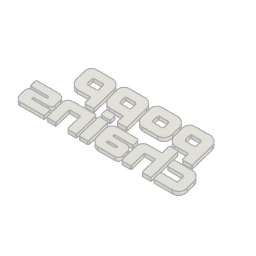
3PoppChains Logo (Autodesk Fusion 360 design; units mm, degrees)
Autodesk Fusion 360 part; units mm, degrees
sketch "PoppChains Logo back" plane through (0, 0, 0) normal (0, 0, 1) x (1, 0, 0)
  line L0 (-12.7934, 7.4385) -> (-14.8073, 7.4385)
  line L1 (-18.0622, -4.0245) -> (-18.1371, -3.7245)
  line L2 (15.775, -3.4869) -> (12.3633, -3.4869)
  line L3 (12.0442, -2.2702) -> (15.4711, -2.2702)
  line L4 (15.4711, -2.2702) -> (15.775, -3.4869)
  arc A0 (11.7104, -2.1972) -> (12.0442, -2.2702) centre (12.0442, -1.4702) ccw
  line L5 (12.0584, -3.5906) -> (11.7104, -2.1972)
  arc A1 (12.3633, -3.4869) -> (12.0584, -3.5906) centre (12.3633, -3.9869) ccw
  spline S0 degree 3 poles (-8.9047, 3.9854) (-8.8081, 3.8641) (-8.7015, 3.7457) (-8.5857, 3.6335) (-8.1655, 3.2264) (-7.6733, 2.9494) (-7.2518, 2.8544) knots 0.109065 0.109065 0.109065 0.109065 0.144103 0.144103 0.144103 0.271229 0.271229 0.271229 0.271229
  spline S1 degree 3 poles (-8.5032, 9.9808) (-9.0129, 9.9808) (-9.5792, 9.7861) (-9.9156, 9.3575) (-10.1073, 9.1132) (-10.2067, 8.8146) (-10.2332, 8.5124) knots 0 0 0 0 0.118832 0.118832 0.118832 0.186572 0.186572 0.186572 0.186572
  spline S2 degree 3 poles (-8.2671, 1.4319) (-8.2484, 1.3571) (-8.211, 1.2855) (-8.27, 1.1136) (-8.3064, 1.0076) (-8.4409, 0.8691) (-8.5685, 0.8357) (-8.6104, 0.8247) (-8.6486, 0.8212) (-8.6817, 0.8212) knots 0 0 0 0 0.007204 0.007204 0.007204 0.011648 0.011648 0.011648 0.01311 0.01311 0.01311 0.01311
  spline S3 degree 2 poles (-12.3757, 7.1783) (-12.4406, 7.4385) (-12.7934, 7.4385) knots 0 0 0 0.053563 0.053563 0.053563 weights 1 1.286007 1
  line L6 (-6.5576, 5.9139) -> (-6.8384, 7.0385)
  line L7 (1.7578, -4.1644) -> (-0.2132, -4.1644)
  arc A2 (-0.4322, -3.9129) -> (-0.2381, -3.6644) centre (-0.2381, -3.8644) cw
  line L8 (-0.4072, -4.0129) -> (-0.4322, -3.9129)
  line L9 (-0.2381, -3.6644) -> (1.7328, -3.6644)
  arc A3 (1.9518, -3.9159) -> (1.7578, -4.1644) centre (1.7578, -3.9644) cw
  arc A4 (-0.2132, -4.1644) -> (-0.4072, -4.0129) centre (-0.2132, -3.9644) cw
  line L10 (1.9268, -3.8159) -> (1.9518, -3.9159)
  arc A5 (1.7328, -3.6644) -> (1.9268, -3.8159) centre (1.7328, -3.8644) cw
  spline S4 degree 2 poles (-16.2032, 9.5808) (-17.8989, 9.5808) (-17.4933, 7.9566) knots 0 0 0 0.236399 0.236399 0.236399 weights 1 0.745447 1
  spline S5 degree 2 poles (-14.3421, 5.4627) (-14.5571, 5.4627) (-14.6454, 5.8161) knots 0 0 0 0.047921 0.047921 0.047921 weights 1 0.521199 1
  arc A6 (-7.2518, 2.8544) -> (-7.4125, 2.3527) centre (-6.9274, 2.4738) ccw
  arc A7 (-4.4905, 5.4627) -> (-4.3062, 5.6987) centre (-4.4905, 5.6527) ccw
  line L11 (-12.4594, 5.8627) -> (-14.2298, 5.8627)
  arc A8 (-11.3768, 3.1416) -> (-11.4739, 3.2173) centre (-11.4739, 3.1173) ccw
  spline S6 degree 2 poles (-20.0623, -2.1426) (-20.9037, -2.1426) (-20.6795, -3.0405) knots 0 0 0 0.121296 0.121296 0.121296 weights 1 0.623284 1
  spline S7 degree 2 poles (-0.9081, 1.3468) (-0.8767, 1.2212) (-0.9817, 1.2212) knots 0 0 0 0.017347 0.017347 0.017347 weights 1 1.074969 1
  spline S8 degree 2 poles (-9.1042, 5.197) (-8.6099, 3.2173) (-6.9332, 3.2173) knots 0 0 0 0.304949 0.304949 0.304949 weights 1 0.564634 1
  line L12 (-2.8716, -6.5063) -> (-4.5755, -6.5063)
  line L13 (-14.6332, 2.8173) -> (-11.7081, 2.8173)
  arc A9 (-6.7172, 0.4953) -> (-6.7594, 0.4425) centre (-6.3489, 0.1571) ccw
  line L14 (-14.2576, 5.9139) -> (-14.5384, 7.0385)
  line L15 (-12.1905, 5.4627) -> (-14.3421, 5.4627)
  line L16 (-12.4594, 5.8627) -> (-12.7528, 7.0377)
  spline S9 degree 3 poles (-12.7528, 7.0377) (-12.7645, 7.0382) (-12.7779, 7.0385) (-12.7934, 7.0385) knots 0.049882 0.049882 0.049882 0.049882 0.053563 0.053563 0.053563 0.053563
  line L17 (-12.0062, 5.6987) -> (-12.3757, 7.1783)
  arc A10 (-8.6888, -1.9459) -> (-8.7858, -1.8702) centre (-8.7858, -1.9702) ccw
  line L18 (-14.6454, 5.8161) -> (-14.9916, 7.2025)
  arc A11 (-16.5004, -2.1426) -> (-16.4034, -2.0184) centre (-16.5004, -2.0426) ccw
  spline S10 degree 3 poles (-0.52, 1.4437) (-0.4968, 1.3508) (-0.4654, 1.2156) (-0.5661, 1.0465) (-0.6478, 0.9093) (-0.8137, 0.8366) (-0.9176, 0.8248) (-0.9404, 0.8222) (-0.9616, 0.8212) (-0.9817, 0.8212) knots 0 0 0 0 0.008721 0.008721 0.008721 0.015794 0.015794 0.015794 0.017347 0.017347 0.017347 0.017347
  spline S11 degree 3 poles (-16.2032, 9.9808) (-16.7129, 9.9808) (-17.2792, 9.7861) (-17.6156, 9.3575) (-17.9484, 8.9335) (-18.0028, 8.3459) (-17.8814, 7.8597) knots 0 0 0 0 0.118832 0.118832 0.118832 0.236399 0.236399 0.236399 0.236399
  line L19 (-2.6776, -5.8579) -> (-4.1289, -0.046)
  line L20 (-6.4459, 0.1329) -> (-4.9636, -5.8032)
  arc A12 (-4.9636, -5.8032) -> (-4.5755, -6.1063) centre (-4.5755, -5.7063) ccw
  arc A13 (-2.8716, -6.1063) -> (-2.6776, -5.8579) centre (-2.8716, -5.9063) ccw
  line L21 (-4.5755, -6.1063) -> (-2.8716, -6.1063)
  arc A14 (-6.3489, 0.2571) -> (-6.4459, 0.1329) centre (-6.3489, 0.1571) ccw
  arc A15 (-4.1289, -0.046) -> (-4.517, 0.2571) centre (-4.517, -0.1429) ccw
  line L22 (-4.517, 0.2571) -> (-6.3489, 0.2571)
  line L23 (-3.2543, -1.367) -> (-2.5651, -4.1266)
  arc A16 (-0.8552, -1.6474) -> (-0.9523, -1.7717) centre (-0.8552, -1.7474) ccw
  spline S12 degree 2 poles (-1.9641, 0.2571) (-3.6598, 0.2571) (-3.2543, -1.367) knots 0 0 0 0.236399 0.236399 0.236399 weights 1 0.745447 1
  spline S13 degree 3 poles (-2.4089, -5.2829) (-2.3011, -5.4235) (-2.18, -5.5609) (-2.0466, -5.6902) (-1.555, -6.1665) (-0.9648, -6.4646) (-0.5045, -6.5018) (-0.4671, -6.5048) (-0.4302, -6.5063) (-0.3941, -6.5063) knots 0.103755 0.103755 0.103755 0.103755 0.144103 0.144103 0.144103 0.292842 0.292842 0.292842 0.304949 0.304949 0.304949 0.304949
  spline S14 degree 3 poles (-10.6898, 0.8212) (-10.9685, 0.8212) (-11.1444, 0.9908) (-11.2604, 1.1724) (-11.2987, 1.2322) (-11.3282, 1.2957) (-11.3458, 1.3662) knots 0 0 0 0 0.028075 0.028075 0.028075 0.037327 0.037327 0.037327 0.037327
  line L24 (-13.7235, -1.3469) -> (-12.6106, -5.8032)
  arc A17 (-20.89, -1.5668) -> (-20.793, -1.6426) centre (-20.793, -1.5426) ccw
  line L25 (-4.7594, 5.8627) -> (-6.5298, 5.8627)
  line L26 (-0.9523, -1.7717) -> (-0.9341, -1.8444)
  arc A18 (-12.6106, -5.8032) -> (-12.2225, -6.1063) centre (-12.2225, -5.7063) ccw
  arc A19 (-2.8716, -6.5063) -> (-2.2895, -5.761) centre (-2.8716, -5.9063) ccw
  arc A20 (-5.5313, -6.5063) -> (-5.1207, -6.2917) centre (-5.5313, -6.0063) ccw
  line L27 (-20.89, -1.5668) -> (-21.3145, 0.1329)
  spline S15 degree 3 poles (-12.5141, 0.6571) (-13.0001, 0.6571) (-13.5417, 0.4643) (-13.8613, 0.0466) (-13.9756, -0.1028) (-14.0554, -0.2722) (-14.1056, -0.4501) knots 0 0 0 0 0.113726 0.113726 0.113726 0.154398 0.154398 0.154398 0.154398
  arc A21 (-11.2381, -1.8702) -> (-11.3352, -1.9944) centre (-11.2381, -1.9702) ccw
  line L28 (-5.0934, 7.0385) -> (-6.8384, 7.0385)
  line L29 (-2.4089, -5.2829) -> (-2.2895, -5.761)
  spline S16 degree 3 poles (-20.7806, -2.0426) (-20.841, -2.1031) (-20.8961, -2.1737) (-20.941, -2.2484) (-21.1119, -2.5324) (-21.1327, -2.8768) (-21.0676, -3.1375) knots 0.049481 0.049481 0.049481 0.049481 0.064439 0.064439 0.064439 0.121296 0.121296 0.121296 0.121296
  line L30 (-13.8926, -2.7331) -> (-14.3478, -0.9104)
  arc A22 (-5.1207, -6.2917) -> (-4.5755, -6.5063) centre (-4.5755, -5.7063) ccw
  line L31 (-17.8814, 7.8597) -> (-17.1923, 5.1001)
  line L32 (-6.9332, 3.2173) -> (-3.7739, 3.2173)
  arc A23 (-13.1783, -6.1063) -> (-13.0813, -5.9821) centre (-13.1783, -6.0063) ccw
  arc A24 (-18.0401, -3.6003) -> (-18.1371, -3.7245) centre (-18.0401, -3.7003) ccw
  arc A25 (-0.9341, -1.8444) -> (-0.546, -2.1474) centre (-0.546, -1.7474) ccw
  line L33 (-5.4343, -5.9821) -> (-6.9166, -0.046)
  arc A26 (-21.2175, 0.2571) -> (-21.3145, 0.1329) centre (-21.2175, 0.1571) ccw
  arc A27 (-13.4755, -4.4033) -> (-13.8636, -4.1003) centre (-13.8636, -4.5003) ccw
  line L34 (-3.7408, 0.0509) -> (-3.6199, -0.4335)
  arc A28 (-21.2175, 0.6571) -> (-21.7026, 0.036) centre (-21.2175, 0.1571) ccw
  line L35 (-13.0813, -5.9821) -> (-13.4755, -4.4033)
  arc A29 (-12.7678, -6.2917) -> (-12.2225, -6.5063) centre (-12.2225, -5.7063) ccw
  line L36 (-5.5313, -6.1063) -> (-7.3375, -6.1063)
  spline S17 degree 2 poles (-2.5651, -4.1266) (-2.0708, -6.1063) (-0.3941, -6.1063) knots 0 0 0 0.304949 0.304949 0.304949 weights 1 0.564634 1
  line L37 (-12.7934, 7.0385) -> (-14.5384, 7.0385)
  arc A30 (-13.1783, -6.5063) -> (-12.7678, -6.2917) centre (-13.1783, -6.0063) ccw
  spline S18 degree 2 poles (-14.3478, -0.9104) (-14.6393, 0.2571) (-15.8774, 0.2571) knots 0 0 0 0.201598 0.201598 0.201598 weights 1 0.666667 1
  line L38 (-16.4783, -1.7184) -> (-16.4034, -2.0184)
  line L39 (8.7039, -2.2702) -> (9.6435, -6.033)
  spline S19 degree 3 poles (7.8687, -5.8354) (7.8948, -5.9397) (7.9271, -6.0356) (7.8693, -6.2046) (7.8256, -6.3322) (7.6744, -6.469) (7.5501, -6.503) (7.4957, -6.5179) (7.4481, -6.5217) (7.4054, -6.5217) knots 0 0 0 0 0.011564 0.011564 0.011564 0.020294 0.020294 0.020294 0.024116 0.024116 0.024116 0.024116
  spline S20 degree 2 poles (6.4947, -1.9838) (6.4663, -1.8702) (6.5435, -1.8702) knots 0 0 0 0.014326 0.014326 0.014326 weights 1 0.986543 1
  line L40 (7.4054, -6.5217) -> (5.4872, -6.5217)
  arc A31 (8.361, 0.2571) -> (8.458, 0.3813) centre (8.361, 0.3571) ccw
  line L41 (6.4947, -1.9838) -> (7.4806, -5.9323)
  arc A32 (9.6435, -6.033) -> (10.2741, -6.5255) centre (10.2741, -5.8755) ccw
  line L42 (9.0447, -1.9838) -> (10.0316, -5.9361)
  spline S21 degree 2 poles (7.4806, -5.9323) (7.528, -6.1217) (7.4054, -6.1217) knots 0 0 0 0.024116 0.024116 0.024116 weights 1 1.205865 1
  line L43 (7.4054, -6.1217) -> (5.4872, -6.1217)
  arc A33 (10.0316, -5.9361) -> (10.2741, -6.1255) centre (10.2741, -5.8755) ccw
  line L44 (6.9784, -2.2702) -> (7.8687, -5.8354)
  spline S22 degree 2 poles (6.4316, 5.2185) (6.9313, 3.2173) (8.5168, 3.2173) knots 0 0 0 0.299728 0.299728 0.299728 weights 1 0.564634 1
  arc A34 (8.3427, 7.4385) -> (8.1584, 7.2025) centre (8.3427, 7.2485) ccw
  line L45 (5.7425, 7.9781) -> (6.4316, 5.2185)
  line L46 (10.3566, 7.0385) -> (8.6116, 7.0385)
  line L47 (10.6906, 5.8627) -> (10.3972, 7.0377)
  spline S23 degree 2 poles (8.8079, 5.4627) (8.5929, 5.4627) (8.5046, 5.8161) knots 0 0 0 0.047921 0.047921 0.047921 weights 1 0.521199 1
  arc A35 (7.8936, 2.9606) -> (7.5515, 2.3603) centre (8.0366, 2.4815) ccw
  line L48 (10.3566, 7.4385) -> (8.3427, 7.4385)
  line L49 (8.0366, 2.5815) -> (9.7924, 2.5815)
  spline S24 degree 3 poles (6.3587, 4.3835) (6.509, 4.1271) (6.7031, 3.8674) (6.9338, 3.6346) (7.2352, 3.3306) (7.5726, 3.0983) (7.8936, 2.9606) knots 0.071956 0.071956 0.071956 0.071956 0.14301 0.14301 0.14301 0.235825 0.235825 0.235825 0.235825
  line L50 (10.6906, 5.8627) -> (8.9202, 5.8627)
  spline S25 degree 2 poles (6.9468, 9.5808) (5.3423, 9.5808) (5.7425, 7.9781) knots 0 0 0 0.228466 0.228466 0.228466 weights 1 0.745447 1
  line L51 (8.8924, 5.9139) -> (8.6116, 7.0385)
  line L52 (8.5046, 5.8161) -> (8.1584, 7.2025)
  arc A36 (10.5686, 2.3753) -> (10.2779, 2.8173) centre (9.7924, 2.1815) ccw
  arc A37 (10.1805, 2.2784) -> (9.7924, 2.5815) centre (9.7924, 2.1815) ccw
  spline S26 degree 3 poles (10.3972, 7.0377) (10.3855, 7.0382) (10.3721, 7.0385) (10.3566, 7.0385) knots 0.049882 0.049882 0.049882 0.049882 0.053563 0.053563 0.053563 0.053563
  spline S27 degree 3 poles (8.9202, 5.8627) (8.9047, 5.885) (8.8943, 5.9083) (8.8924, 5.9139) knots 0.029456 0.029456 0.029456 0.029456 0.044721 0.044721 0.044721 0.044721
  spline S28 degree 3 poles (6.3587, 4.3835) (6.3212, 4.0569) (6.2153, 3.7527) (6.0237, 3.4998) (5.6676, 3.0297) (5.0602, 2.8173) (4.4476, 2.8173) knots 0.078476 0.078476 0.078476 0.078476 0.154724 0.154724 0.154724 0.296505 0.296505 0.296505 0.296505
  spline S29 degree 5 poles (5.2144, 0.2571) (5.2086, 0.2571) (5.1964, 0.2572) (5.1763, 0.2578) (5.1458, 0.2592) (5.102, 0.2605) (5.0526, 0.2596) (4.9982, 0.2548) (4.9395, 0.2452) (4.8777, 0.2304) (4.814, 0.2108) (4.7496, 0.1869) (4.6858, 0.1592) (4.6237, 0.1283) (4.5643, 0.0946) (4.5084, 0.0584) (4.4562, 0.0199) (4.4081, -0.0207) (4.3635, -0.0634) (4.322, -0.1081) (4.2826, -0.1547) (4.2448, -0.2031) (4.208, -0.2532) (4.1726, -0.3046) (4.1391, -0.3569) (4.1084, -0.41) (4.0813, -0.4637) (4.0585, -0.5181) (4.0402, -0.5741) (4.0259, -0.6327) (4.0151, -0.6948) (4.0071, -0.7616) (4.0011, -0.8333) (3.9969, -0.9096) (3.9941, -0.9893) (3.9929, -1.071) (3.9934, -1.153) (3.9957, -1.2334) (4, -1.311) (4.0064, -1.3848) (4.0151, -1.4543) (4.0237, -1.5063) (4.0313, -1.5432) (4.0367, -1.5669) (4.0395, -1.5785) knots 0 0 0 0 0 0 0.025 0.05 0.075 0.1 0.125 0.15 0.175 0.2 0.225 0.25 0.275 0.3 0.325 0.35 0.375 0.4 0.425 0.45 0.475 0.5 0.525 0.55 0.575 0.6 0.625 0.65 0.675 0.7 0.725 0.75 0.775 0.8 0.825 0.85 0.875 0.9 0.925 0.95 0.975 1 1 1 1 1 1
  spline S30 degree 2 poles (5.3449, 7.5066) (4.8269, 9.5808) (2.9577, 9.5808) knots 0 0 0 0.329195 0.329195 0.329195 weights 1 0.594055 1
  spline S31 degree 3 poles (5.2144, 0.6571) (5.186, 0.6571) (4.889, 0.6635) (4.6506, 0.5763) (4.3416, 0.4633) (4.0734, 0.2363) (3.9128, 0.0202) (3.8114, -0.1163) (3.7062, -0.2874) (3.6522, -0.4818) knots 0 0 0 0 0.210086 0.210086 0.210086 0.482519 0.482519 0.482519 0.654552 0.654552 0.654552 0.654552
  spline S32 degree 3 poles (6.9468, 9.9808) (6.4622, 9.9808) (5.9221, 9.788) (5.6036, 9.371) (5.4157, 9.1249) (5.3212, 8.8246) (5.2988, 8.5214) knots 0 0 0 0 0.113417 0.113417 0.113417 0.18033 0.18033 0.18033 0.18033
  line L53 (7.9769, 0.6571) -> (7.5515, 2.3603)
  spline S33 degree 2 poles (5.8873, 5.3346) (6.416, 3.2173) (4.4476, 3.2173) knots 0 0 0 0.296505 0.296505 0.296505 weights 1 0.847333 1
  line L54 (10.6577, 9.9808) -> (6.9468, 9.9808)
  line L55 (5.8873, 5.3346) -> (5.3449, 7.5066)
  spline S34 degree 3 poles (5.2988, 8.5214) (5.1508, 8.7377) (4.9713, 8.9504) (4.7641, 9.1433) (4.2375, 9.6337) (3.5919, 9.9356) (3.0894, 9.9755) (3.0445, 9.979) (3.0006, 9.9808) (2.9577, 9.9808) knots 0.091726 0.091726 0.091726 0.091726 0.154738 0.154738 0.154738 0.314905 0.314905 0.314905 0.329195 0.329195 0.329195 0.329195
  arc A38 (4.711, -5.9157) -> (5.4872, -6.5217) centre (5.4872, -5.7217) ccw
  arc A39 (8.0366, 2.5815) -> (7.9396, 2.4572) centre (8.0366, 2.4815) ccw
  line L56 (10.6577, 9.5808) -> (6.9468, 9.5808)
  line L57 (8.458, 0.3813) -> (7.9396, 2.4572)
  line L58 (4.0395, -1.5785) -> (5.0991, -5.8187)
  line L59 (3.5001, -1.5232) -> (3.1688, -0.1974)
  spline S35 degree 3 poles (2.6972, 7.0377) (2.6855, 7.0382) (2.6721, 7.0385) (2.6566, 7.0385) knots 0.049882 0.049882 0.049882 0.049882 0.053563 0.053563 0.053563 0.053563
  spline S36 degree 2 poles (1.1079, 5.4627) (0.8929, 5.4627) (0.8046, 5.8161) knots 0 0 0 0.047921 0.047921 0.047921 weights 1 0.521199 1
  arc A40 (0.6427, 7.4385) -> (0.4584, 7.2025) centre (0.6427, 7.2485) ccw
  line L60 (3.6522, -0.4818) -> (3.5569, -0.1005)
  spline S37 degree 3 poles (1.2202, 5.8627) (1.2048, 5.8848) (1.1941, 5.9087) (1.1924, 5.9139) knots 0.029456 0.029456 0.029456 0.029456 0.044721 0.044721 0.044721 0.044721
  line L61 (2.6566, 7.0385) -> (0.9116, 7.0385)
  spline S38 degree 3 poles (4.6962, -5.8563) (4.6582, -5.9337) (4.6125, -6.0075) (4.5584, -6.0759) (4.3359, -6.3574) (3.9893, -6.5063) (3.6964, -6.5063) knots 0.072101 0.072101 0.072101 0.072101 0.088502 0.088502 0.088502 0.156035 0.156035 0.156035 0.156035
  line L62 (2.6566, 7.4385) -> (0.6427, 7.4385)
  line L63 (3.4438, 5.6987) -> (3.0743, 7.1783)
  line L64 (0.8046, 5.8161) -> (0.4584, 7.2025)
  arc A41 (3.2595, 5.4627) -> (3.4438, 5.6987) centre (3.2595, 5.6527) ccw
  line L65 (2.5867, 0.6571) -> (-1.9641, 0.6571)
  line L66 (4.0361, -3.3747) -> (4.4167, -4.8975)
  line L67 (1.1924, 5.9139) -> (0.9116, 7.0385)
  line L68 (4.6962, -5.8563) -> (4.711, -5.9157)
  spline S39 degree 2 poles (3.0743, 7.1783) (3.0094, 7.4385) (2.6566, 7.4385) knots 0 0 0 0.053563 0.053563 0.053563 weights 1 1.286007 1
  spline S40 degree 2 poles (4.4167, -4.8975) (4.7187, -6.1063) (3.6964, -6.1063) knots 0 0 0 0.156035 0.156035 0.156035 weights 1 0.619231 1
  line L69 (3.2595, 5.4627) -> (1.1079, 5.4627)
  arc A42 (3.4031, -1.6474) -> (3.5001, -1.5232) centre (3.4031, -1.5474) ccw
  line L70 (2.9906, 5.8627) -> (2.6972, 7.0377)
  arc A43 (3.1688, -0.1974) -> (2.5867, 0.2571) centre (2.5867, -0.3429) ccw
  line L71 (2.9906, 5.8627) -> (1.2202, 5.8627)
  arc A44 (3.5569, -0.1005) -> (2.5867, 0.6571) centre (2.5867, -0.3429) ccw
  spline S41 degree 2 poles (4.0361, -3.3747) (3.7295, -2.1474) (2.492, -2.1474) knots 0 0 0 0.204563 0.204563 0.204563 weights 1 0.543429 1
  line L72 (0.8168, 2.8173) -> (4.4476, 2.8173)
  line L73 (0.8168, 3.2173) -> (4.4476, 3.2173)
  line L74 (8.7039, -2.2702) -> (6.9784, -2.2702)
  line L75 (7.9769, 0.6571) -> (5.2144, 0.6571)
  arc A45 (9.0447, -1.9838) -> (8.8991, -1.8702) centre (8.8991, -2.0202) ccw
  arc A46 (5.0991, -5.8187) -> (5.4872, -6.1217) centre (5.4872, -5.7217) ccw
  line L76 (8.361, 0.2571) -> (5.2144, 0.2571)
  line L77 (8.8991, -1.8702) -> (6.5435, -1.8702)
  line L78 (-4.0081, 2.8173) -> (-3.6458, 1.3662)
  line L79 (15.8592, -2.1733) -> (16.2561, -3.7627)
  arc A47 (11.6561, -1.5671) -> (12.0442, -1.8702) centre (12.0442, -1.4702) ccw
  line L80 (19.0529, -3.9076) -> (18.5105, -1.7355)
  line L81 (13.0276, -6.5217) -> (17.2251, -6.5217)
  line L82 (12.2662, -4.0112) -> (12.7365, -5.8944)
  arc A48 (12.7789, -6.4761) -> (13.0276, -6.5217) centre (13.0276, -5.8217) ccw
  line L83 (18.6648, -4.0045) -> (18.1224, -1.8324)
  arc A49 (15.8592, -2.1733) -> (15.4711, -1.8702) centre (15.4711, -2.2702) ccw
  spline S42 degree 2 poles (18.6648, -4.0045) (19.1935, -6.1217) (17.2251, -6.1217) knots 0 0 0 0.296505 0.296505 0.296505 weights 1 0.847333 1
  line L84 (2.9577, 9.5808) -> (-0.7532, 9.5808)
  line L85 (2.5867, 0.2571) -> (-1.9641, 0.2571)
  line L86 (-0.3941, -6.1063) -> (3.6964, -6.1063)
  line L87 (-0.3941, -6.5063) -> (3.6964, -6.5063)
  line L88 (2.9577, 9.9808) -> (-0.7532, 9.9808)
  line L89 (16.1591, -3.8869) -> (12.3633, -3.8869)
  spline S43 degree 3 poles (-1.1547, 3.9854) (-1.0581, 3.8641) (-0.9515, 3.7457) (-0.8357, 3.6335) (-0.3441, 3.1571) (0.2461, 2.8591) (0.7064, 2.8219) (0.7439, 2.8188) (0.7807, 2.8173) (0.8168, 2.8173) knots 0.109065 0.109065 0.109065 0.109065 0.144103 0.144103 0.144103 0.292842 0.292842 0.292842 0.304949 0.304949 0.304949 0.304949
  line L90 (3.4031, -1.6474) -> (-0.8552, -1.6474)
  line L91 (-0.546, -2.1474) -> (2.492, -2.1474)
  spline S44 degree 3 poles (14.9754, 1.455) (15.0011, 1.3519) (15.0173, 1.1877) (14.9096, 1.0322) (14.8062, 0.8828) (14.6427, 0.8346) (14.5375, 0.8244) (14.5134, 0.8221) (14.4906, 0.8212) (14.4683, 0.8212) knots 0 0 0 0 0.00997 0.00997 0.00997 0.019549 0.019549 0.019549 0.021738 0.021738 0.021738 0.021738
  line L92 (15.7352, 0.2571) -> (11.3286, 0.2571)
  line L93 (11.4419, 2.8173) -> (11.8042, 1.3662)
  spline S45 degree 3 poles (13.4396, 7.6052) (13.3215, 8.078) (12.979, 8.6704) (12.4693, 9.1437) (11.9418, 9.6334) (11.2948, 9.9351) (10.7915, 9.9753) (10.7459, 9.979) (10.7013, 9.9808) (10.6577, 9.9808) knots 0 0 0 0 0.154866 0.154866 0.154866 0.315107 0.315107 0.315107 0.329614 0.329614 0.329614 0.329614
  line L94 (-5.0934, 7.4385) -> (-7.1073, 7.4385)
  line L95 (-13.1783, -6.1063) -> (-18.8142, -6.1063)
  spline S46 degree 3 poles (-14.1056, -0.4501) (-14.286, -0.1199) (-14.5902, 0.2021) (-14.9542, 0.4037) (-15.2635, 0.575) (-15.5944, 0.6571) (-15.8774, 0.6571) knots 0.03353 0.03353 0.03353 0.03353 0.124381 0.124381 0.124381 0.201598 0.201598 0.201598 0.201598
  arc A50 (-5.5313, -6.1063) -> (-5.4343, -5.9821) centre (-5.5313, -6.0063) ccw
  line L96 (14.9754, 1.455) -> (13.4396, 7.6052)
  line L97 (-12.4923, 9.5808) -> (-16.2032, 9.5808)
  spline S47 degree 2 poles (-16.8042, 5.197) (-16.3099, 3.2173) (-14.6332, 3.2173) knots 0 0 0 0.304949 0.304949 0.304949 weights 1 0.564634 1
  arc A51 (11.3286, 0.6571) -> (11.0236, 0.5532) centre (11.3286, 0.1571) ccw
  spline S48 degree 2 poles (-1.3542, 5.197) (-0.8599, 3.2173) (0.8168, 3.2173) knots 0 0 0 0.304949 0.304949 0.304949 weights 1 0.564634 1
  line L98 (-10.4364, -6.5063) -> (-12.2225, -6.5063)
  spline S49 degree 3 poles (-10.2332, 8.5124) (-10.3777, 8.7302) (-10.5523, 8.9447) (-10.7532, 9.1391) (-11.2695, 9.6389) (-11.8986, 9.9446) (-12.3914, 9.9774) (-12.4256, 9.9796) (-12.4593, 9.9808) (-12.4923, 9.9808) knots 0.091177 0.091177 0.091177 0.091177 0.153242 0.153242 0.153242 0.312762 0.312762 0.312762 0.323826 0.323826 0.323826 0.323826
  line L99 (15.7352, 0.6571) -> (11.3286, 0.6571)
  line L100 (-7.3047, 0.6571) -> (-12.5141, 0.6571)
  spline S50 degree 2 poles (-12.5141, 0.2571) (-14.124, 0.2571) (-13.7235, -1.3469) knots 0 0 0 0.228928 0.228928 0.228928 weights 1 0.745447 1
  line L101 (14.4683, 0.8212) -> (12.4602, 0.8212)
  line L102 (10.2779, 2.8173) -> (11.4419, 2.8173)
  line L103 (14.5873, 1.3581) -> (13.0515, 7.5083)
  line L104 (12.2791, -6.1255) -> (10.1805, 2.2784)
  line L105 (12.2791, -6.1255) -> (10.2741, -6.1255)
  line L106 (-10.3394, -5.9821) -> (-11.3352, -1.9944)
  spline S51 degree 2 poles (13.0515, 7.5083) (12.534, 9.5808) (10.6577, 9.5808) knots 0 0 0 0.329614 0.329614 0.329614 weights 1 0.594055 1
  line L107 (11.2316, 0.1329) -> (11.6561, -1.5671)
  line L108 (-9.0201, -2.2702) -> (-10.854, -2.2702)
  line L109 (-10.4364, -6.1063) -> (-12.2225, -6.1063)
  spline S52 degree 2 poles (-10.191, 7.4852) (-10.7143, 9.5808) (-12.4923, 9.5808) knots 0 0 0 0.323826 0.323826 0.323826 weights 1 0.594055 1
  line L110 (8.5168, 3.2173) -> (11.6761, 3.2173)
  line L111 (-4.7923, 9.9808) -> (-8.5032, 9.9808)
  spline S53 degree 2 poles (12.4602, 1.2212) (12.2527, 1.2212) (12.1923, 1.4631) knots 0 0 0 0.037327 0.037327 0.037327 weights 1 0.521007 1
  line L112 (-15.8774, 0.6571) -> (-21.2175, 0.6571)
  line L113 (-8.7858, -1.8702) -> (-11.2381, -1.8702)
  line L114 (14.4683, 1.2212) -> (12.4602, 1.2212)
  spline S54 degree 2 poles (10.7743, 7.1783) (10.7094, 7.4385) (10.3566, 7.4385) knots 0 0 0 0.053563 0.053563 0.053563 weights 1 1.286007 1
  line L115 (-6.6817, 1.077) -> (-7.0244, 2.4496)
  line L116 (-6.9274, 2.5738) -> (-5.0955, 2.5738)
  arc A52 (-7.0244, 2.4496) -> (-6.9274, 2.5738) centre (-6.9274, 2.4738) cw
  arc A53 (-6.2936, 0.7739) -> (-6.6817, 1.077) centre (-6.2936, 1.1739) cw
  line L117 (-4.7074, 2.2707) -> (-4.3647, 0.8981)
  arc A54 (-4.3647, 0.8981) -> (-4.4617, 0.7739) centre (-4.4617, 0.8739) cw
  line L118 (-4.4617, 0.7739) -> (-6.2936, 0.7739)
  arc A55 (-5.0955, 2.5738) -> (-4.7074, 2.2707) centre (-5.0955, 2.1738) cw
  arc A56 (10.9595, 5.4627) -> (11.1438, 5.6987) centre (10.9595, 5.6527) ccw
  line L119 (-7.3047, 0.2571) -> (-12.5141, 0.2571)
  line L120 (-12.4923, 9.9808) -> (-16.2032, 9.9808)
  spline S55 degree 3 poles (-17.1923, 5.1001) (-17.0828, 4.6617) (-16.762, 4.095) (-16.2857, 3.6335) (-15.7941, 3.1571) (-15.2039, 2.8591) (-14.7436, 2.8219) (-14.7061, 2.8188) (-14.6693, 2.8173) (-14.6332, 2.8173) knots 0 0 0 0 0.144103 0.144103 0.144103 0.292842 0.292842 0.292842 0.304949 0.304949 0.304949 0.304949
  line L121 (-15.8774, 0.2571) -> (-21.2175, 0.2571)
  line L122 (10.9595, 5.4627) -> (8.8079, 5.4627)
  arc A57 (11.7732, 3.1416) -> (11.6761, 3.2173) centre (11.6761, 3.1173) ccw
  line L123 (-4.7923, 9.5808) -> (-8.5032, 9.5808)
  line L124 (11.1438, 5.6987) -> (10.7743, 7.1783)
  line L125 (-4.4905, 5.4627) -> (-6.6421, 5.4627)
  line L126 (11.0236, 0.5532) -> (10.5686, 2.3753)
  line L127 (-9.9513, -5.8852) -> (-10.854, -2.2702)
  line L128 (-8.6817, 1.2212) -> (-10.6898, 1.2212)
  line L129 (-13.8636, -4.1003) -> (-17.9652, -4.1003)
  line L130 (-14.6171, -3.6003) -> (-18.0401, -3.6003)
  spline S56 degree 3 poles (12.4602, 0.8212) (12.1815, 0.8212) (12.0056, 0.9908) (11.8896, 1.1724) (11.8513, 1.2322) (11.8218, 1.2957) (11.8042, 1.3662) knots 0 0 0 0 0.028075 0.028075 0.028075 0.037327 0.037327 0.037327 0.037327
  line L131 (12.7912, -6.5255) -> (10.2741, -6.5255)
  line L132 (-8.6817, 0.8212) -> (-10.6898, 0.8212)
  spline S57 degree 2 poles (14.5873, 1.3581) (14.6215, 1.2212) (14.4683, 1.2212) knots 0 0 0 0.021738 0.021738 0.021738 weights 1 1.074969 1
  spline S58 degree 2 poles (18.1224, -1.8324) (17.6006, 0.2571) (15.7352, 0.2571) knots 0 0 0 0.330226 0.330226 0.330226 weights 1 0.594055 1
  spline S59 degree 3 poles (18.5105, -1.7355) (18.392, -1.2609) (18.0505, -0.6648) (17.5426, -0.1879) (17.0164, 0.3061) (16.3711, 0.6111) (15.8681, 0.6517) (15.8229, 0.6553) (15.7786, 0.6571) (15.7352, 0.6571) knots 0 0 0 0 0.155097 0.155097 0.155097 0.315776 0.315776 0.315776 0.330226 0.330226 0.330226 0.330226
  arc A58 (11.3286, 0.2571) -> (11.2316, 0.1329) centre (11.3286, 0.1571) ccw
  line L133 (11.7732, 3.1416) -> (12.1923, 1.4631)
  line L134 (-5.5313, -6.5063) -> (-7.3375, -6.5063)
  line L135 (-13.1783, -6.5063) -> (-18.8142, -6.5063)
  spline S60 degree 2 poles (-14.6171, -3.6003) (-13.6761, -3.6003) (-13.8926, -2.7331) knots 0 0 0 0.126916 0.126916 0.126916 weights 1 0.666667 1
  arc A59 (16.1591, -3.8869) -> (16.2561, -3.7627) centre (16.1591, -3.7869) ccw
  line L136 (13.0276, -6.1217) -> (17.2251, -6.1217)
  line L137 (12.0442, -1.8702) -> (15.4711, -1.8702)
  line L138 (12.7912, -6.5255) -> (12.7789, -6.4761)
  arc A60 (12.7365, -5.8944) -> (13.0276, -6.1217) centre (13.0276, -5.8217) ccw
  arc A61 (12.3633, -3.8869) -> (12.2662, -4.0112) centre (12.3633, -3.9869) ccw
  spline S61 degree 3 poles (19.0529, -3.9076) (19.2262, -4.6014) (19.19, -5.3262) (18.8013, -5.8393) (18.4451, -6.3094) (17.8378, -6.5217) (17.2251, -6.5217) knots 0 0 0 0 0.154724 0.154724 0.154724 0.296505 0.296505 0.296505 0.296505
  line L139 (-16.5754, -1.6426) -> (-20.793, -1.6426)
  line L140 (-21.2781, -1.6637) -> (-21.7026, 0.036)
  spline S62 degree 2 poles (-4.6757, 7.1783) (-4.7406, 7.4385) (-5.0934, 7.4385) knots 0 0 0 0.053563 0.053563 0.053563 weights 1 1.286007 1
  arc A62 (-12.1905, 5.4627) -> (-12.0062, 5.6987) centre (-12.1905, 5.6527) ccw
  spline S63 degree 2 poles (-6.6421, 5.4627) (-6.8571, 5.4627) (-6.9454, 5.8161) knots 0 0 0 0.047921 0.047921 0.047921 weights 1 0.521199 1
  line L141 (-0.9817, 1.2212) -> (-2.9898, 1.2212)
  line L142 (-0.52, 1.4437) -> (-1.1547, 3.9854)
  line L143 (-20.6223, -4.9208) -> (-21.0676, -3.1375)
  spline S64 degree 2 poles (-8.6552, 1.335) (-8.6267, 1.2212) (-8.6817, 1.2212) knots 0 0 0 0.01311 0.01311 0.01311 weights 1 1.074969 1
  arc A63 (-10.4364, -6.5063) -> (-9.9513, -5.8852) centre (-10.4364, -6.0063) ccw
  arc A64 (-14.8073, 7.4385) -> (-14.9916, 7.2025) centre (-14.8073, 7.2485) ccw
  line L144 (-16.5004, -2.1426) -> (-20.0623, -2.1426)
  line L145 (-11.3768, 3.1416) -> (-10.9577, 1.4631)
  spline S65 degree 3 poles (-5.0528, 7.0377) (-5.0645, 7.0382) (-5.0779, 7.0385) (-5.0934, 7.0385) knots 0.049882 0.049882 0.049882 0.049882 0.053563 0.053563 0.053563 0.053563
  arc A65 (-10.4364, -6.1063) -> (-10.3394, -5.9821) centre (-10.4364, -6.0063) ccw
  line L146 (-8.2671, 1.4319) -> (-8.9047, 3.9854)
  spline S66 degree 3 poles (-0.7532, 9.9808) (-1.2629, 9.9808) (-1.8292, 9.7861) (-2.1656, 9.3575) (-2.3578, 9.1126) (-2.4572, 8.8131) (-2.4834, 8.5101) knots 0 0 0 0 0.118832 0.118832 0.118832 0.186742 0.186742 0.186742 0.186742
  spline S67 degree 2 poles (-2.9898, 1.2212) (-3.1973, 1.2212) (-3.2577, 1.4631) knots 0 0 0 0.037327 0.037327 0.037327 weights 1 0.521007 1
  arc A66 (-3.6768, 3.1416) -> (-3.7739, 3.2173) centre (-3.7739, 3.1173) ccw
  line L147 (-8.1137, -5.9001) -> (-9.0201, -2.2702)
  line L148 (-3.6768, 3.1416) -> (-3.2577, 1.4631)
  spline S68 degree 2 poles (-2.4439, 7.497) (-2.9643, 9.5808) (-4.7923, 9.5808) knots 0 0 0 0.326756 0.326756 0.326756 weights 1 0.594055 1
  spline S69 degree 3 poles (-6.5298, 5.8627) (-6.5453, 5.885) (-6.5557, 5.9083) (-6.5576, 5.9139) knots 0.029456 0.029456 0.029456 0.029456 0.044721 0.044721 0.044721 0.044721
  line L149 (-2.0433, 7.9566) -> (-1.3542, 5.197)
  arc A67 (-6.7594, 0.4425) -> (-7.3047, 0.6571) centre (-7.3047, -0.1429) ccw
  spline S70 degree 2 poles (-8.5032, 9.5808) (-10.1989, 9.5808) (-9.7933, 7.9566) knots 0 0 0 0.236399 0.236399 0.236399 weights 1 0.745447 1
  line L150 (-20.2342, -4.8239) -> (-20.6795, -3.0405)
  line L151 (-7.0697, 0.9801) -> (-7.4125, 2.3527)
  arc A68 (-16.4783, -1.7184) -> (-16.5754, -1.6426) centre (-16.5754, -1.7426) ccw
  line L152 (-11.7081, 2.8173) -> (-11.3458, 1.3662)
  spline S71 degree 3 poles (-14.2298, 5.8627) (-14.2453, 5.885) (-14.2557, 5.9083) (-14.2576, 5.9139) knots 0.029456 0.029456 0.029456 0.029456 0.044721 0.044721 0.044721 0.044721
  spline S72 degree 3 poles (-2.9898, 0.8212) (-3.2685, 0.8212) (-3.4444, 0.9908) (-3.5604, 1.1724) (-3.5987, 1.2322) (-3.6282, 1.2957) (-3.6458, 1.3662) knots 0 0 0 0 0.028075 0.028075 0.028075 0.037327 0.037327 0.037327 0.037327
  arc A69 (-8.1137, -5.9001) -> (-7.3375, -6.5063) centre (-7.3375, -5.7063) ccw
  line L153 (-17.4933, 7.9566) -> (-16.8042, 5.197)
  line L154 (-9.7933, 7.9566) -> (-9.1042, 5.197)
  line L155 (-4.3062, 5.6987) -> (-4.6757, 7.1783)
  line L156 (-14.6332, 3.2173) -> (-11.4739, 3.2173)
  arc A70 (-3.7408, 0.0509) -> (-4.0934, 0.5357) centre (-4.517, -0.1429) ccw
  line L157 (-4.3194, 2.3677) -> (-3.9766, 0.995)
  spline S73 degree 2 poles (-0.7532, 9.5808) (-2.4489, 9.5808) (-2.0433, 7.9566) knots 0 0 0 0.236399 0.236399 0.236399 weights 1 0.745447 1
  line L158 (-20.7806, -2.0426) -> (-20.793, -2.0426)
  arc A71 (-7.1073, 7.4385) -> (-7.2916, 7.2025) centre (-7.1073, 7.2485) ccw
  line L159 (-0.9081, 1.3468) -> (-2.4439, 7.497)
  arc A72 (-18.0622, -4.0245) -> (-17.9652, -4.1003) centre (-17.9652, -4.0003) ccw
  arc A73 (-4.3194, 2.3677) -> (-4.6203, 2.8173) centre (-5.0955, 2.1738) ccw
  spline S74 degree 3 poles (-18.8142, -6.5063) (-19.2524, -6.5063) (-19.8041, -6.2103) (-20.1761, -5.7665) (-20.4048, -5.4935) (-20.5555, -5.1883) (-20.6223, -4.9208) knots 0 0 0 0 0.12361 0.12361 0.12361 0.199614 0.199614 0.199614 0.199614
  line L160 (-4.7594, 5.8627) -> (-5.0528, 7.0377)
  arc A74 (-21.2781, -1.6637) -> (-20.793, -2.0426) centre (-20.793, -1.5426) ccw
  line L161 (-6.9454, 5.8161) -> (-7.2916, 7.2025)
  spline S75 degree 2 poles (-18.8142, -6.1063) (-19.9139, -6.1063) (-20.2342, -4.8239) knots 0 0 0 0.199614 0.199614 0.199614 weights 1 0.626857 1
  spline S76 degree 2 poles (-10.6898, 1.2212) (-10.8973, 1.2212) (-10.9577, 1.4631) knots 0 0 0 0.037327 0.037327 0.037327 weights 1 0.521007 1
  spline S77 degree 3 poles (-2.4834, 8.5101) (-2.6307, 8.7295) (-2.8096, 8.9454) (-3.016, 9.1411) (-3.5378, 9.6356) (-4.1758, 9.9393) (-4.6737, 9.9763) (-4.714, 9.9793) (-4.7536, 9.9808) (-4.7923, 9.9808) knots 0.090787 0.090787 0.090787 0.090787 0.154026 0.154026 0.154026 0.313823 0.313823 0.313823 0.326756 0.326756 0.326756 0.326756
  arc A75 (-4.0934, 0.5357) -> (-3.9766, 0.995) centre (-4.4617, 0.8739) ccw
  line L162 (-0.9817, 0.8212) -> (-2.9898, 0.8212)
  arc A76 (-7.0697, 0.9801) -> (-6.7172, 0.4953) centre (-6.2936, 1.1739) ccw
  arc A77 (-6.9166, -0.046) -> (-7.3047, 0.2571) centre (-7.3047, -0.1429) ccw
  line L163 (-7.7256, -5.8032) -> (-8.6888, -1.9459)
  line L164 (-8.6552, 1.335) -> (-10.191, 7.4852)
  line L165 (-4.6203, 2.8173) -> (-4.0081, 2.8173)
  spline S78 degree 3 poles (-1.9641, 0.6571) (-2.4739, 0.6571) (-3.0401, 0.4624) (-3.3765, 0.0338) (-3.4871, -0.1071) (-3.567, -0.2662) (-3.6199, -0.4335) knots 0 0 0 0 0.118832 0.118832 0.118832 0.157913 0.157913 0.157913 0.157913
  arc A78 (-7.7256, -5.8032) -> (-7.3375, -6.1063) centre (-7.3375, -5.7063) ccw
sketch "Sketch2 offset outer shape" plane through (0, 0, 0) normal (0, 0, 1) x (1, 0, 0)
  line L0 (14.9754, 1.455) -> (13.4396, 7.6052) construction
  spline S0 degree 3 poles (13.4396, 7.6052) (13.3215, 8.078) (12.979, 8.6704) (12.4693, 9.1437) (11.9418, 9.6334) (11.2948, 9.9351) (10.7915, 9.9753) (10.7459, 9.979) (10.7013, 9.9808) (10.6577, 9.9808) knots 0 0 0 0 0.154866 0.154866 0.154866 0.315107 0.315107 0.315107 0.329614 0.329614 0.329614 0.329614
  line L1 (10.6577, 9.9808) -> (6.9468, 9.9808) construction
  line L2 (-12.4923, 9.9808) -> (-16.2032, 9.9808) construction
  spline S1 degree 3 poles (-16.2032, 9.9808) (-16.7129, 9.9808) (-17.2792, 9.7861) (-17.6156, 9.3575) (-17.9484, 8.9335) (-18.0028, 8.3459) (-17.8814, 7.8597) knots 0 0 0 0 0.118832 0.118832 0.118832 0.236399 0.236399 0.236399 0.236399
  line L3 (-17.8814, 7.8597) -> (-17.1923, 5.1001) construction
  arc A0 (-21.2175, 0.6571) -> (-21.7026, 0.036) centre (-21.2175, 0.1571) ccw construction
  line L4 (-20.6223, -4.9208) -> (-21.0676, -3.1375) construction
  spline S2 degree 3 poles (-18.8142, -6.5063) (-19.2524, -6.5063) (-19.8041, -6.2103) (-20.1761, -5.7665) (-20.4048, -5.4935) (-20.5555, -5.1883) (-20.6223, -4.9208) knots 0 0 0 0 0.12361 0.12361 0.12361 0.199614 0.199614 0.199614 0.199614
  line L5 (-13.1783, -6.5063) -> (-18.8142, -6.5063) construction
  line L6 (13.0276, -6.5217) -> (17.2251, -6.5217) construction
  spline S3 degree 3 poles (19.0529, -3.9076) (19.2262, -4.6014) (19.19, -5.3262) (18.8013, -5.8393) (18.4451, -6.3094) (17.8378, -6.5217) (17.2251, -6.5217) knots 0 0 0 0 0.154724 0.154724 0.154724 0.296505 0.296505 0.296505 0.296505
  line L7 (19.0529, -3.9076) -> (18.5105, -1.7355) construction
  spline S4 degree 3 poles (18.5105, -1.7355) (18.392, -1.2609) (18.0505, -0.6648) (17.5426, -0.1879) (17.0164, 0.3061) (16.3711, 0.6111) (15.8681, 0.6517) (15.8229, 0.6553) (15.7786, 0.6571) (15.7352, 0.6571) knots 0 0 0 0 0.155097 0.155097 0.155097 0.315776 0.315776 0.315776 0.330226 0.330226 0.330226 0.330226
  spline S5 degree 5 poles (15.7352, 0.6571) (15.6802, 0.6571) (15.5768, 0.6665) (15.4412, 0.7086) (15.2949, 0.8132) (15.1538, 0.9973) (15.0669, 1.1702) (15.0155, 1.3093) (14.9877, 1.4058) (14.9754, 1.455) knots 0 0 0 0 0 0 0.2 0.4 0.6 0.8 1 1 1 1 1 1
  spline S6 degree 5 poles (6.9468, 9.9808) (6.1692, 9.9808) (4.6141, 9.9808) (2.2814, 9.9808) (-0.8289, 9.9808) (-4.7167, 9.9808) (-7.827, 9.9808) (-10.1597, 9.9808) (-11.7148, 9.9808) (-12.4923, 9.9808) knots 0 0 0 0 0 0 0.2 0.4 0.6 0.8 1 1 1 1 1 1
  spline S7 degree 5 poles (-21.0676, -3.1375) (-21.099, -3.0118) (-21.1587, -2.7597) (-21.2391, -2.3798) (-21.3316, -1.8702) (-21.4385, -1.2313) (-21.531, -0.7217) (-21.6115, -0.3418) (-21.6712, -0.0897) (-21.7026, 0.036) knots 0 0 0 0 0 0 0.2 0.4 0.6 0.8 1 1 1 1 1 1
  spline S8 degree 5 poles (13.0276, -6.5217) (11.9793, -6.5217) (9.8829, -6.5214) (6.7382, -6.52) (2.5452, -6.5166) (-2.696, -6.5115) (-6.8889, -6.508) (-10.0336, -6.5066) (-12.1301, -6.5063) (-13.1783, -6.5063) knots 0 0 0 0 0 0 0.2 0.4 0.6 0.8 1 1 1 1 1 1
  line L8 (-17.1923, 5.1001) -> (-16.2186, 1.2008) construction
  line L9 (-21.2175, 0.6571) -> (-16.7054, 0.6571) construction
  spline S9 degree 5 poles (-16.2186, 1.2008) (-16.2089, 1.1621) (-16.1977, 1.0879) (-16.2054, 0.9863) (-16.258, 0.8687) (-16.3729, 0.752) (-16.4919, 0.6882) (-16.5938, 0.6628) (-16.6673, 0.6571) (-16.7054, 0.6571) knots 0 0 0 0 0 0 0.2 0.4 0.6 0.8 1 1 1 1 1 1
  spline S10 degree 5 poles (15.3327, 1.6749) (15.3402, 1.6451) (15.3554, 1.584) (15.3791, 1.4875) (15.4142, 1.353) (15.4748, 1.1965) (15.5505, 1.1034) (15.6317, 1.0655) (15.6986, 1.0571) (15.7352, 1.0571) knots 0 0 0 0 0 0 0.2 0.4 0.6 0.8 1 1 1 1 1 1
  spline S11 degree 5 poles (-16.6942, 1.4544) (-16.6886, 1.4322) (-16.681, 1.3877) (-16.68, 1.3215) (-16.6973, 1.2352) (-16.7455, 1.1398) (-16.805, 1.0845) (-16.8638, 1.0621) (-16.9099, 1.0571) (-16.9348, 1.0571) knots 0 0 0 0 0 0 0.2 0.4 0.6 0.8 1 1 1 1 1 1
  line L10 (-16.6942, 1.4544) -> (-17.5804, 5.0032)
  line L11 (-17.5804, 5.0032) -> (-16.6067, 1.1039) construction
  spline S12 degree 3 poles (-16.6067, 1.1039) (-16.6059, 1.1008) (-16.6053, 1.0982) (-16.605, 1.0961) knots 0 0 0 0 0.034557 0.034557 0.034557 0.034557
  spline S13 degree 3 poles (-16.605, 1.0961) (-16.6136, 1.0861) (-16.6409, 1.0571) (-16.7054, 1.0571) knots 0.463709 0.463709 0.463709 0.463709 1 1 1 1
  line L12 (-21.2175, 1.0571) -> (-16.7054, 1.0571)
  arc A1 (-21.2175, 1.0571) -> (-22.0907, -0.061) centre (-21.2175, 0.1571) ccw
  spline S14 degree 3 poles (-21.4557, -3.2344) (-21.725, -2.1557) (-21.8369, -1.0773) (-22.0907, -0.061) knots 0 0 0 0 1 1 1 1
  line L13 (-21.0103, -5.0177) -> (-21.4557, -3.2344)
  spline S15 degree 3 poles (-18.8142, -6.9063) (-19.4325, -6.9063) (-20.0418, -6.5494) (-20.4826, -6.0234) (-20.7501, -5.7042) (-20.9266, -5.353) (-21.0103, -5.0177) knots 0 0 0 0 0.12361 0.12361 0.12361 0.199614 0.199614 0.199614 0.199614
  line L14 (-13.1783, -6.9063) -> (-18.8142, -6.9063)
  spline S16 degree 3 poles (13.0276, -6.9217) (4.2919, -6.9217) (-4.4434, -6.9063) (-13.1783, -6.9063) knots 0 0 0 0 1 1 1 1
  line L15 (13.0276, -6.9217) -> (17.2251, -6.9217)
  spline S17 degree 3 poles (19.441, -3.8107) (19.6333, -4.5807) (19.6111, -5.4327) (19.1201, -6.0808) (18.6668, -6.6792) (17.9302, -6.9217) (17.2251, -6.9217) knots 0 0 0 0 0.154724 0.154724 0.154724 0.296505 0.296505 0.296505 0.296505
  line L16 (19.441, -3.8107) -> (18.8986, -1.6386)
  spline S18 degree 3 poles (18.8986, -1.6386) (18.7554, -1.0652) (18.3804, -0.4258) (17.8164, 0.1037) (17.2311, 0.6532) (16.5361, 0.9991) (15.9003, 1.0504) (15.8446, 1.0549) (15.7896, 1.0571) (15.7352, 1.0571) knots 0 0 0 0 0.155097 0.155097 0.155097 0.315776 0.315776 0.315776 0.330226 0.330226 0.330226 0.330226
  spline S19 degree 3 poles (15.7352, 1.0571) (15.6253, 1.0571) (15.6161, 1.0719) (15.5519, 1.1476) (15.4812, 1.231) (15.4051, 1.385) (15.3635, 1.5519) knots 0 0 0 0 0.475568 0.475568 0.475568 1 1 1 1
  line L17 (15.3635, 1.5519) -> (13.8276, 7.7021)
  spline S20 degree 3 poles (13.8276, 7.7021) (13.6846, 8.2751) (13.3077, 8.9111) (12.7414, 9.4369) (12.1544, 9.9818) (11.4578, 10.3233) (10.8234, 10.3741) (10.7674, 10.3785) (10.7122, 10.3808) (10.6577, 10.3808) knots 0 0 0 0 0.154866 0.154866 0.154866 0.315107 0.315107 0.315107 0.329614 0.329614 0.329614 0.329614
  line L18 (10.6577, 10.3808) -> (6.9468, 10.3808)
  spline S21 degree 1 poles (6.9468, 10.3808) (-12.4923, 10.3808) knots 0 0 1.943912 1.943912
  line L19 (-12.4923, 10.3808) -> (-16.2032, 10.3808)
  spline S22 degree 3 poles (-16.2032, 10.3808) (-16.8148, 10.3808) (-17.4956, 10.1582) (-17.9302, 9.6044) (-18.3607, 9.0559) (-18.4161, 8.3498) (-18.2695, 7.7628) knots 0 0 0 0 0.118832 0.118832 0.118832 0.236399 0.236399 0.236399 0.236399
  line L20 (-18.2695, 7.7628) -> (-17.5804, 5.0032)
  dimension "d1" = -0.4
  constraint coincident S4.end S5.start
  constraint coincident L0.start S5.end
  constraint coincident L1.end S6.start
  constraint coincident L2.start S6.end
  constraint coincident L4.end S7.start
  constraint coincident A0.end S7.end
  constraint tangent A0 S7
  constraint coincident L6.start S8.start
  constraint coincident L5.start S8.end
  constraint coincident L3.end L8.start
  constraint parallel L3 L8
  constraint coincident A0.start L9.start
  constraint tangent A0 L9
  constraint coincident S10.start L17
  constraint coincident S11.start L11
  constraint coincident S11.end L12
extrude "White Letters - Extrude3" add sketch "PoppChains Logo back" along normal blind 0.8 contours L1 S6 A11 A17 L27 L30 A23 A24 A26 A27 L35 S18 L38 L95 L121 L129 L130 S60 L139 L144 L150 A68 A72 S75 | S4 A8 L97 S47 S52 L128 S64 L145 L153 L156 S76 L164 | S7 S8 L32 L123 L141 S67 A66 L148 S68 S70 L154 L159 | A10 L24 A18 A21 L33 L36 A50 S50 L106 L109 L113 L119 A65 A77 L163 A78 | L19 L20 A12 A13 L21 A14 A15 L22 | L23 A16 S12 L26 A25 S17 L59 L66 S40 A42 A43 S41 L85 L86 L90 L91 | S20 A31 L41 L42 S21 L43 A33 L49 A37 S29 A39 L57 L58 A45 A46 L76 L77 L104 L105 | S22 L45 S25 L56 L103 S51 L110 S53 L114 A57 S57 L133 | S30 S33 L55 L73 L84 S48 L149 S73 | L79 A47 L82 L83 A49 S42 L89 L92 L107 S58 A58 A59 L136 L137 A60 A61 | L115 L116 A52 A53 L117 A54 L118 A55 makes body 1 at (1.6867, -5.459, 0) makes body 2 at (-7.0132, -2.658, 0) makes body 3 at (13.1348, 4.0095, 0) makes body 4 at (-10.0769, 3.9942, 0) makes body 5 at (-5.1795, -1.9055, 0) makes body 6 at (10.5014, -1.9437, 0) makes body 7 at (-16.6526, -5.4376, 0) makes body 8 at (2.8413, 3.9658, 0) makes body 9 at (-2.3455, 4.002, 0) makes body 10 at (-6.2349, 2.0749, 0) makes body 11 at (15.4706, -5.3768, 0)
extrude "Negative - Extrude5" add sketch "PoppChains Logo back" along normal blind 0.4 separate body makes body 12 at (-5.2973, 5.596, 0) makes body 13 at (8.782, 2.7934, 0) makes body 14 at (-12.9973, 5.596, 0) makes body 15 at (2.4527, 5.596, 0) makes body 16 at (10.1527, 5.596, 0) makes body 17 at (1.0925, -3.9977, 0)
copy_body "CopyPasteBodies2" bodies 1 2 3 4 5 6 7 8 9 10 11 makes body 18 makes body 19 makes body 20 makes body 21 makes body 22 makes body 23 makes body 24 makes body 25 makes body 26 makes body 27 makes body 28
combine "negative bodies - Combine2" operation add target body 12 tool bodies 13 26 25 24 14 17 16 15 28 18 27 19 20 21 22 23
named bodies: "White PC letters 7 a", "White PC letters 10 n", "White PC letters 1 p", "White PC letters 4 p", "White PC letters 8 i", "White PC letters 6 h", "White PC letters 11 s", "White PC letters 2 o", "White PC letters 3 p", "White PC letters 9 i dot", "White PC letters 5 c", "TOOL - subtract from base - NEGATIVE", "White PC letters 7 a (1)", "White PC letters 10 n (1)", "White PC letters 1 p (1)", "White PC letters 4 p (1)", "White PC letters 8 i (1)", "White PC letters 6 h (1)", "White PC letters 11 s (1)", "White PC letters 2 o (1)", "White PC letters 3 p (1)", "White PC letters 9 i dot (1)", "White PC letters 5 c (1)"
